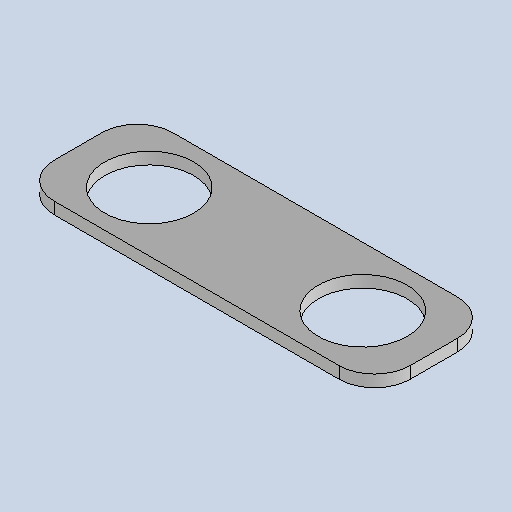
# Autodesk Inventor part: motor pillar 2
Saved by Autodesk Inventor 2025.3 (Build 293356030, 356C)
## iProperties
Created: 2025-09-03
Part Number: motor pillar 2
Material: Generic
Document SubType Name: Sheet Metal
Designer: admin
Density: 1 g/cm^3
Sheet Metal Rule: Default
Appearance: Default
Mass: 1.63134 g
Surface Area: 21.1923 cm^2
Volume: 1.63134 cm^3
Flat Pattern Width: 2 cm
Flat Pattern Length: 6 cm
Flat Pattern Area: 12 cm^2
Sheet Metal Width: 20,000 mm
Sheet Metal Length: 60,000 mm
Sheet Metal Area: 1200,000 mm^2
Author: admin
Autodesk Inventor part; units mm, degrees
ref_plane "YZ Plane" through (0, 0, 0) normal (1, 0, 0) x (0, 1, 0)
ref_plane "XZ Plane" through (0, 0, 0) normal (0, 1, 0) x (-1, 0, 0)
ref_plane "XY Plane" through (0, 0, 0) normal (0, 0, 1) x (1, 0, 0)
sketch "Sketch1" plane through (0, 0, 0) normal (0, 0, 1) x (1, 0, 0)
  line L0 (-30, 10) -> (30, 10)
  line L1 (30, 10) -> (30, -10)
  line L2 (30, -10) -> (-30, -10)
  line L3 (-30, -10) -> (-30, 10)
  line L4 (-30, 10) -> (30, -10) construction
  line L5 (30, 10) -> (-30, -10) construction
  circle A0 centre (18, 0) radius 7.5
  circle A1 centre (-18, 0) radius 7.5
  line L6 (0, 10) -> (0, -10) construction
  point P0 (0, 0)
  point P1 (0, 0)
  dimension "d0" = 60
  dimension "d1" = 20
  dimension "d2" = 15
  dimension "d3" = 36
  measures "d0" distance of L1.end L2.end
  measures "d1" distance of L0.end L1.end
  measures "d2" diameter of A1
  measures "d3" distance of A0.centre A1.centre
extrude "Plate1" add sketch "Sketch1" along normal blind 2
fillet "Corner Round1" radius 6 4 edges at (-30, 10, 1) (-30, -10, 1) (30, 10, 1) (30, -10, 1)
equation "\"d4\" = Thickness"
equation "\"BendRadius\" = Thickness"
equation "\"BendReliefWidth\" = Thickness"
equation "\"BendReliefDepth\" = 0.5 * Thickness"
equation "\"CornerReliefSize\" = 4 * Thickness"
equation "\"MinimumRemnant\" = 2 * Thickness"
equation "\"TransitionRadius\" = BendRadius"
equation "\"JacobiRadiusSize\" = BendRadius"
equation "\"GapSize\" = Thickness"
equation "\"Thickness\" = 2"
body "Solid1"
